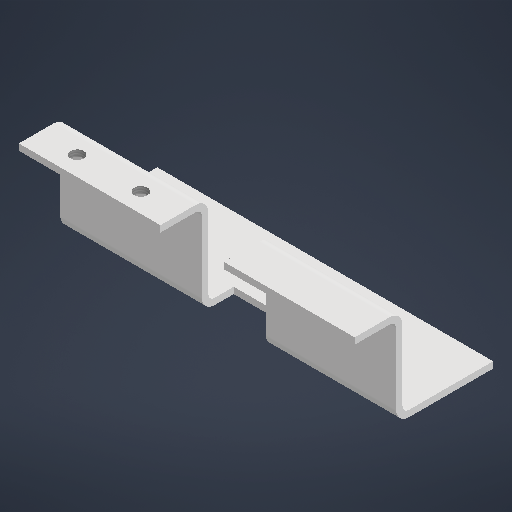
# Autodesk Inventor part: Bottom joint housing 2R
Saved by Autodesk Inventor 2026.3 (Build 303398000, 398)
## iProperties
Created: 2026-08-05
Part Number: Bottom joint housing 2R
Material: Generic
Document SubType Name: Sheet Metal
Designer: matot
Density: 1 g/cm^3
Sheet Metal Rule: Default_mm
Appearance: Default
Author: matot
Autodesk Inventor part; units mm, degrees
ref_plane "YZ Plane" through (0, 0, 0) normal (1, 0, 0) x (0, 1, 0)
ref_plane "XZ Plane" through (0, 0, 0) normal (0, 1, 0) x (-1, 0, 0)
ref_plane "XY Plane" through (0, 0, 0) normal (0, 0, 1) x (1, 0, 0)
sketch "Sketch1" plane through (0, 0, 0) normal (0, 1, 0) x (-1, 0, 0)
  line L0 (171.8333, 340.8333) -> (-39.1667, 340.8333)
  line L1 (-39.1667, 340.8333) -> (-39.1667, -59.1667)
  line L2 (-39.1667, -59.1667) -> (171.8333, -59.1667)
  line L3 (171.8333, -59.1667) -> (171.8333, 340.8333)
  point P0 (0, 0)
  dimension "d0" = 400
  dimension "d1" = 211
  measures "d0" distance of L0.end L1.end
  measures "d1" distance of L1.end L2.end
extrude "Plate1" add sketch "Sketch1" along normal blind 4
sketch "Sketch2" plane through (0, 4, 0) normal (0, 1, 0) x (1, 0, 0)
  line L0 (-171.8333, 59.1667) -> (-171.8333, -340.8333) projected
  line L1 (-171.8333, -137.1069) -> (39.1667, -137.1069)
  line L2 (-171.8333, -37.1069) -> (39.1667, -37.1069)
  line L3 (39.1667, -37.1069) -> (39.1667, -37.1069)
  line L4 (39.1667, 59.1667) -> (39.1667, -340.8333) projected
  point P0 (0, 0)
  dimension "d3" = 100
  dimension "d4" = 211
  dimension "d5" = 211
  constraints: 6 end point, 3 perpendicular, 2 point on line, 1 horizontal
  measures "d3" distance between parallel lines of L2 L1
  measures "d4" distance of L2.start L2.end
  measures "d5" distance of L1.start L1.end
fold "Fold1" angle 90 bend radius 4 thickness 4 k factor 0.44 line from (-171.8333, 4, 37.1069) to (39.1667, 4, 37.1069) line at bend centre moving side (0, 0, -1) folds toward (0, 1, 0)
sketch "Sketch3" plane through (0, 0, 0) normal (0, -1, 0) x (1, 0, 0)
  line L0 (39.1667, 41.6308) -> (39.1667, 340.8333) projected
  line L1 (39.1667, 90.6308) -> (-171.8333, 90.6308)
  line L2 (39.1667, 33.6308) -> (-171.8333, 33.6308) projected
  point P0 (0, 0)
  dimension "d12" = 211
  dimension "d13" = 57
  constraints: 2 end point, 1 horizontal, 1 point on line
  measures "d12" distance of L1.start L1.end
  measures "d13" distance between parallel lines of L2 L1
fold "Fold2" angle 90 bend radius 4 thickness 4 k factor 0.44 line from (39.1667, 0, 90.6308) to (-171.8333, 0, 90.6308) line at bend centre moving side (0, 0, -1) folds toward (0, -1, 0)
sketch "Sketch4" plane through (0, 4, 0) normal (0, 1, 0) x (1, 0, 0)
  line L0 (-171.8333, -340.8333) -> (-171.8333, -95.1547) projected
  line L1 (-171.8333, -117.1547) -> (39.1667, -117.1547)
  line L2 (-171.8333, -87.1547) -> (39.1667, -87.1547) projected
  line L3 (39.1667, -95.1547) -> (39.1667, -340.8333) projected
  line L4 (39.1667, -117.1547) -> (-171.8333, -117.1547)
  line L5 (-171.8333, -117.1547) -> (-171.8333, -340.8333)
  line L6 (-171.8333, -340.8333) -> (39.1667, -340.8333)
  line L7 (39.1667, -340.8333) -> (39.1667, -117.1547)
  point P0 (0, 0)
  point P1 (-66.3333, -87.1547)
  dimension "d20" = 211
  dimension "d21" = 30
  constraints: 10 end point, 2 horizontal, 2 parallel, 2 perpendicular, 1 midpoint, 1 point on line
  measures "d20" distance of L1.start L1.end
  measures "d21" distance from line of point (-66.333, -87.155) L1
extrude "Cut1" cut sketch "Sketch4" against normal through all
sketch "Sketch5" plane through (-171.8333, -56.4761, -8.595) normal (0, -1, 0) x (1, 0, 0)
  line L0 (0, 0) -> (0, 91.7497) projected
  line L1 (0, 38.7497) -> (211, 38.7497)
  line L2 (0, 99.7497) -> (211, 99.7497) projected
  line L3 (211, 91.7497) -> (211, 0) projected
  line L4 (211, 0) -> (0, 0) projected
  line L5 (211, 38.7497) -> (0, 38.7497)
  line L6 (0, 38.7497) -> (0, 0)
  line L7 (0, 0) -> (211, 0)
  line L8 (211, 0) -> (211, 38.7497)
  point P0 (171.8333, 8.595)
  dimension "d24" = 211
  dimension "d25" = 61
  constraints: 10 end point, 2 horizontal, 2 parallel, 2 perpendicular, 1 point on line
  measures "d24" distance of L1.start L1.end
  measures "d25" distance between parallel lines of L2 L1
extrude "Cut2" cut sketch "Sketch5" against normal through all
sketch "Sketch6" plane through (-171.8333, -48.4761, 91.1547) normal (0, 0, 1) x (1, 0, 0)
  line L0 (211, 52.4761) -> (0, 52.4761) projected
  line L1 (211, -8) -> (0, -8) projected
  line L2 (89, 52.4761) -> (129, 52.4761)
  line L3 (129, 52.4761) -> (129, -8)
  line L4 (129, -8) -> (89, -8)
  line L5 (89, -8) -> (89, 52.4761)
  line L6 (0, 0) -> (0, 44.4761) projected
  line L7 (89, -8) -> (129, -8)
  line L8 (129, -8) -> (129, 52.4761)
  line L9 (129, 52.4761) -> (89, 52.4761)
  line L10 (89, 52.4761) -> (89, -8)
  point P0 (171.8333, 48.4761)
  point P1 (129, 22.2381)
  point P2 (89, 22.2381)
  point P3 (89, -8)
  point P4 (129, 52.4761)
  dimension "d28" = 40
  dimension "d29" = 89
  constraints: 16 end point, 4 parallel, 2 horizontal, 2 midpoint, 2 perpendicular, 2 point on line
  measures "d28" distance of point (129, 22.238) point (89, 22.238)
  measures "d29" distance between parallel lines of L6 L5
extrude "Cut3" cut sketch "Sketch6" along normal through all
sketch "Sketch7" plane through (-171.8333, -48.4761, 91.1547) normal (0, 0, 1) x (1, 0, 0)
  line L0 (89, 52.4761) -> (0, 52.4761) projected
  line L1 (211, -8) -> (0, -8) projected
  line L2 (89, 52.4761) -> (129, 52.4761)
  line L3 (129, 52.4761) -> (129, -8)
  line L4 (129, -8) -> (89, -8)
  line L5 (89, -8) -> (89, 52.4761)
  point P0 (171.8333, 48.4761)
  point P1 (89, -8)
  constraints: 8 end point, 2 parallel, 1 horizontal, 1 perpendicular, 1 point on line
extrude "Cut4" cut sketch "Sketch7" against normal blind 20
sketch "Sketch8" plane through (-171.8333, -56.4761, 30.1547) normal (0, -1, 0) x (1, 0, 0)
  line L0 (0, 0) -> (211, 0) projected
  line L1 (211, 53) -> (211, 0) projected
  point P0 (171.8333, -30.1547)
  point P1 (145, 26.75)
  point P2 (73.8, 26.75)
  point P3 (211, 26.5)
  dimension "d34" = 26.75
  dimension "d35" = 66
  dimension "d36" = 26.75
  dimension "d37" = 71.2
  constraints: 1 midpoint
  measures "d34" distance from line of point (145, 26.75) L0
  measures "d35" horizontal distance of point (211, 26.5) point (145, 26.75)
  measures "d36" distance from line of L0 point (73.8, 26.75)
  measures "d37" distance of point (145, 26.75) point (73.8, 26.75)
hole "Hole1" at (-26.8333, -56.4761, 56.9047) at (-98.0333, -56.4761, 56.9047) direction (0, 1, 0) diameter 3.242 depth 11.8 tip angle 118 thread size "M4x0.7" class "6H" standard "ISO Metric profile"
sketch "Sketch9" plane through (-171.8333, -56.4761, 30.1547) normal (0, -1, 0) x (1, 0, 0)
  line L0 (0, 0) -> (211, 0) projected
  circle A0 centre (145, 26.75) radius 1.621 projected
  point P0 (171.8333, -30.1547)
  point P1 (126.9, 17.5)
  point P2 (91.9, 17.5)
  dimension "d45" = 17.5
  dimension "d46" = 17.5
  dimension "d47" = 35
  dimension "d48" = 18.1
  measures "d45" distance from line of L0 point (126.9, 17.5)
  measures "d46" distance from line of L0 point (91.9, 17.5)
  measures "d47" distance of point (91.9, 17.5) point (126.9, 17.5)
  measures "d48" horizontal distance of A0.centre point (126.9, 17.5)
hole "Hole2" at (-44.9333, -56.4761, 47.6547) at (-79.9333, -56.4761, 47.6547) direction (0, 1, 0) diameter 3.242 end through all thread size "M4x0.7" class "6H" standard "ISO Metric profile"
sketch "Sketch10" plane through (0, 4, 0) normal (0, 1, 0) x (1, 0, 0)
  line L0 (-171.8333, -117.1547) -> (-82.8333, -117.1547) projected
  line L1 (-171.8333, -117.1547) -> (-171.8333, -95.1547) projected
  point P0 (0, 0)
  point P1 (-147.3333, -105)
  point P2 (-107.3333, -105)
  dimension "d56" = 12.1547
  dimension "d57" = 12.1547
  dimension "d58" = 40
  dimension "d59" = 24.5
  measures "d56" distance from line of L0 point (-147.333, -105)
  measures "d57" distance from line of L0 point (-107.333, -105)
  measures "d58" distance of point (-107.333, -105) point (-147.333, -105)
  measures "d59" distance from line of L1 point (-147.333, -105)
hole "Hole3" at (-147.3333, 4, 105) at (-107.3333, 4, 105) direction (0, -1, 0) diameter 8.376 end through all thread size "M10x1.5" class "6H" standard "ISO Metric profile"
equation "\"d2\" = Thickness"
equation "\"d6\" = BendReliefWidth"
equation "\"d7\" = BendReliefDepth"
equation "\"d8\" = MinimumRemnant"
equation "\"d9\" = TransitionRadius"
equation "\"d11\" = BendRadius"
equation "\"d14\" = BendReliefWidth"
equation "\"d15\" = BendReliefDepth"
equation "\"d16\" = MinimumRemnant"
equation "\"d17\" = TransitionRadius"
equation "\"d19\" = BendRadius"
equation "\"d22\" = Thickness"
equation "\"d26\" = Thickness"
equation "\"d30\" = Thickness"
equation "\"d54\" = Thickness"
equation "\"d65\" = Thickness"
equation "\"BendRadius\" = Thickness"
equation "\"BendReliefWidth\" = Thickness"
equation "\"BendReliefDepth\" = 0.5 * Thickness"
equation "\"CornerReliefSize\" = 4 * Thickness"
equation "\"MinimumRemnant\" = 2 * Thickness"
equation "\"TransitionRadius\" = BendRadius"
equation "\"JacobiRadiusSize\" = BendRadius"
equation "\"GapSize\" = Thickness"
equation "\"Thickness\" = 4"
body "Solid1"
